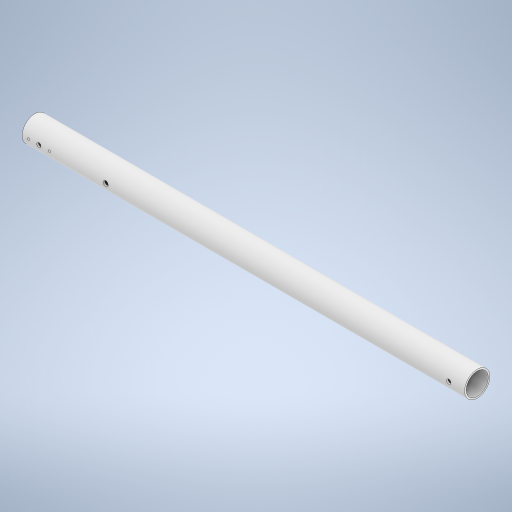
# Autodesk Inventor part: Arm Segment 1
Saved by Autodesk Inventor 2023 (Build 270158030, 158C)
## iProperties
Created: 2022-10-01
Part Number: Arm Segment 1
Material: PVC-Piping
Document SubType Name: Modeling
Designer: cjj5381
Density: 1.4 g/cm^3
Appearance: Smooth - White
Author: cjj5381
Autodesk Inventor part; units mm, degrees
ref_plane "YZ Plane" through (0, 0, 0) normal (1, 0, 0) x (0, 1, 0)
ref_plane "XZ Plane" through (0, 0, 0) normal (0, 1, 0) x (-1, 0, 0)
ref_plane "XY Plane" through (0, 0, 0) normal (0, 0, 1) x (1, 0, 0)
sketch "Sketch1" plane through (0, 0, 0) normal (1, 0, 0) x (0, 1, 0)
  circle A0 centre (0, 0) radius 26.2509
  circle A1 centre (0, 0) radius 30.1625
  dimension "d0" = 52.5018
  dimension "d1" = 3.9116
  constraints: 2 centre point, 1 coincident
  measures "d0" diameter of A0
  measures "d1" radial gap between concentric circles of A0 A1
extrude "Extrusion1" add sketch "Sketch1" along normal mid plane 1060
sketch "Sketch3" plane through (0, 0, 0) normal (0, 0, 1) x (1, 0, 0)
  circle A0 centre (491.9, 0) radius 5.25
  line L0 (530, 26.2509) -> (530, -26.2509) projected
  point P0 (0, 0)
  dimension "d8" = 10.5
  dimension "d9" = 38.1
  constraints: 1 centre point
  measures "d8" diameter of A0
  measures "d9" distance from line of L0 A0.centre
extrude "Extrusion3" cut sketch "Sketch3" along normal through all both and the other way through all
sketch "Sketch5" plane through (0, 0, 0) normal (0, 0, 1) x (1, 0, 0)
  circle A0 centre (-330, 0) radius 6
  line L0 (-530, -26.2509) -> (-530, 26.2509) projected
  point P0 (0, 0)
  dimension "d17" = 12
  dimension "d18" = 200
  constraints: 1 centre point
  measures "d17" diameter of A0
  measures "d18" distance from line of L0 A0.centre
extrude "Extrusion5" cut sketch "Sketch5" along normal through all both and the other way through all
sketch "Sketch6" plane through (0, 0, 0) normal (0, 0, 1) x (1, 0, 0)
  circle A0 centre (-490, 0) radius 5
  line L0 (-530, -26.2509) -> (-530, 26.2509) projected
  circle A1 centre (-515, 0) radius 2.5
  circle A2 centre (-465, 0) radius 2.5
  line L1 (-490, 0) -> (-490, 42.8638) construction
  point P0 (0, 0)
  dimension "d21" = 10
  dimension "d22" = 40
  dimension "d25" = 50
  dimension "d26" = 5
  constraints: 3 centre point, 2 end point, 1 equal radius, 1 symmetric about line, 1 vertical
  measures "d21" diameter of A0
  measures "d22" distance from line of L0 L1.start
  measures "d25" distance of A2.centre A1.centre
  measures "d26" diameter of A1
extrude "Extrusion6" cut sketch "Sketch6" along normal through all both and the other way through all
body "Solid1"
